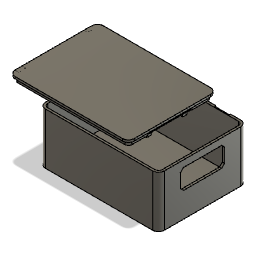
public-monitor-bridge-case (Autodesk Fusion 360 design; units mm, degrees)
Autodesk Fusion 360 part; units mm, degrees
note: some values were not read from the file. Set by a fixed rule: which face or edge a step refers to.
sketch "Base" plane through (0, 0, 0) normal (0, 1, 0) x (1, 0, 0) in component "Top"
  line L0 (0, 0) -> (81, 0)
  line L1 (81, 0) -> (81, 60)
  line L2 (81, 60) -> (0, 60)
  line L3 (0, 60) -> (0, 0)
  dimension "d6" = 81
  dimension "d7" = 60
  constraint horizontal L0
  constraint vertical L1
  constraint horizontal L2
  constraint vertical L3
  constraint coincident L0.start L3.end
  measures "d6" distance of L0.start L0.end
  measures "d7" distance of L0.start L2.end
extrude "Extrude1" add sketch "Base" along normal blind 35 makes body 1 in component "Top"
fillet "Fillet1" radius 4 4 edges at (81, 17.5, 0) (0, 17.5, 0) (81, 17.5, -60) (0, 17.5, -60) on bodies 1 in component "Top"
shell "Shell1" thickness 1.5 removed faces 1 at (52.6667, 35, -20) on bodies 1 in component "Top"
sketch "Knob" plane through (1.5, 0, 0) normal (1, 0, 0) x (0, 0, -1) in component "Top"
  line L0 (56, 1.5) -> (56, 35)
  line L1 (56, 35) -> (4, 35)
  line L2 (4, 35) -> (4, 1.5)
  line L3 (4, 1.5) -> (56, 1.5)
  line L4 (15, 35) -> (45, 35)
  line L5 (45, 35) -> (45, 32)
  line L6 (45, 32) -> (15, 32)
  line L7 (15, 32) -> (15, 35)
  line L8 (30, 35) -> (30, 32) construction
  dimension "d12" = 30
  dimension "d13" = 3
  constraint horizontal L4
  constraint vertical L5
  constraint horizontal L6
  constraint vertical L7
  constraint coincident L1 L4.start
  constraint midpoint L1 L8.start
  constraint midpoint L6 L8.end
  constraint vertical L8
  measures "d12" distance of L5.end L6.end
  measures "d13" distance of L4.end L5.end
extrude "Extrude2" add sketch "Knob" along normal blind 6 draft -45 contours L1 L4 L5 L6 L7 bodies 1 in component "Top"
ref_plane "WorkPlane2" through (40.5, 17.5, -30) normal (-1, 0, 0) x (0, 0, 1) in component "Top"
mirror "Mirror1" about plane through (40.5, 17.5, -30) normal (-1, 0, 0) of "Extrude2" in component "Top"
sketch "Top" plane through (0, 35, 0) normal (0, 1, 0) x (-1, 0, 0) in component "Base"
  line L0 (-81, -4) -> (-81, -56)
  arc A0 (-81, -56) -> (-77, -60) centre (-77, -56) ccw
  line L1 (-77, -60) -> (-4, -60)
  arc A1 (-4, -60) -> (0, -56) centre (-4, -56) ccw
  line L2 (0, -56) -> (0, -4)
  arc A2 (0, -4) -> (-4, 0) centre (-4, -4) ccw
  line L3 (-4, 0) -> (-77, 0)
  arc A3 (-77, 0) -> (-81, -4) centre (-77, -4) ccw
  line L4 (-79.5, -15) -> (-79.5, -4)
  arc A4 (-77, -1.5) -> (-79.5, -4) centre (-77, -4) ccw
  line L5 (-77, -1.5) -> (-4, -1.5)
  arc A5 (-1.5, -4) -> (-4, -1.5) centre (-4, -4) ccw
  line L6 (-1.5, -4) -> (-1.5, -15)
  line L7 (-1.5, -15) -> (-1.5, -45)
  line L8 (-1.5, -45) -> (-1.5, -56)
  arc A6 (-4, -58.5) -> (-1.5, -56) centre (-4, -56) ccw
  line L9 (-4, -58.5) -> (-77, -58.5)
  arc A7 (-79.5, -56) -> (-77, -58.5) centre (-77, -56) ccw
  line L10 (-79.5, -56) -> (-79.5, -45)
  line L11 (-79.5, -45) -> (-79.5, -15)
extrude "Extrude1'" add sketch "Top" along normal blind 1.5 separate body contours L0 A0 L1 A1 L2 A2 L3 A3 | L4 A4 L5 A5 L6 L7 L8 A6 L9 A7 L10 L11 makes body 2 in component "Base"
sketch "Lip" plane through (0, 35, 0) normal (0, -1, 0) x (1, 0, 0) in component "Base"
  arc A0 (81, -4) -> (77, 0) centre (77, -4) ccw
  line L0 (77, 0) -> (4, 0)
  arc A1 (4, 0) -> (0, -4) centre (4, -4) ccw
  line L1 (0, -4) -> (0, -56)
  arc A2 (0, -56) -> (4, -60) centre (4, -56) ccw
  line L2 (4, -60) -> (77, -60)
  arc A3 (77, -60) -> (81, -56) centre (77, -56) ccw
  line L3 (81, -56) -> (81, -4)
  line L4 (79.3, -56) -> (79.3, -4)
  arc A4 (79.3, -4) -> (77, -1.7) centre (77, -4) ccw
  line L5 (77, -1.7) -> (4, -1.7)
  arc A5 (4, -1.7) -> (1.7, -4) centre (4, -4) ccw
  line L6 (1.7, -4) -> (1.7, -56)
  arc A6 (1.7, -56) -> (4, -58.3) centre (4, -56) ccw
  line L7 (4, -58.3) -> (77, -58.3)
  arc A7 (77, -58.3) -> (79.3, -56) centre (77, -56) ccw
  dimension "d19" = 1.7
extrude "Extrude2'" add sketch "Lip" along normal blind 3 contours L4 A4 L5 A5 L6 A6 L7 A7 bodies 2 in component "Base"
extrude "Extrude3" cut sketch "Knob" along normal blind 3 draft -45 from surface at 0.2 contours L1 L4 L5 L6 L7 bodies 2 in component "Base"
mirror "Mirror1'" about plane through (40.5, 17.5, -30) normal (-1, 0, 0) of "Extrude3" in component "Base"
shell "Shell1'" thickness 1.5 removed faces 1 at (27.5667, 32, -35) on bodies 2 in component "Base"
chamfer "Chamfer1" distance 0.6 angle 45 2 edges at (1.7, 32, -30) (79.3, 32, -30) on bodies 2 in component "Base"
sketch "ttl-cutout" plane through (81, 0, 0) normal (1, 0, 0) x (0, 0, -1) in component "Top"
  line L0 (56, 35) -> (4, 35)
  line L1 (4, 35) -> (4, 0)
  line L2 (4, 0) -> (56, 0)
  line L3 (56, 0) -> (56, 35)
  line L4 (0, 35) -> (0, 0)
  line L5 (0, 0) -> (60, 0)
  line L6 (15, 35) -> (45, 35)
  line L7 (45, 35) -> (45, 17)
  line L8 (45, 17) -> (15, 17)
  line L9 (15, 17) -> (15, 35)
  line L10 (30, 35) -> (30, 0) construction
  line L11 (45, 35) -> (43.5, 33.5) construction
  line L12 (43.5, 33.5) -> (16.5, 33.5) construction
  line L13 (16.5, 33.5) -> (15, 35) construction
  line L14 (15, 35) -> (45, 35) construction
  line L15 (15, 32) -> (16.5, 33.5) construction
  line L16 (16.5, 33.5) -> (43.5, 33.5) construction
  line L17 (43.5, 33.5) -> (45, 32) construction
  line L18 (45, 32) -> (15, 32) construction
  line L19 (15, 30.5) -> (45, 30.5)
  point P0 (30, 17)
  point P1 (30, 35)
  dimension "d73" = 30
  dimension "d74" = 18
  dimension "d75" = 1.5
  constraint horizontal L6
  constraint vertical L7
  constraint horizontal L8
  constraint vertical L9
  constraint coincident L0 L6.start
  constraint midpoint L8 P0
  constraint midpoint L0 P1
  constraint coincident P1 L10.start
  constraint midpoint L2 L10.end
  constraint coincident P0 L10
  constraint coincident L9 L19.start
  constraint coincident L7 L19.end
  constraint perpendicular L7 L19
  measures "d73" distance of L6.start L6.end
  measures "d74" distance of L6.start L8.end
  measures "d75" distance of L18 L19
sketch "pcb-mount" plane through (12.1976, 35, -8.3625) normal (0, -1, 0) x (1, 0, 0) in component "Base"
  line L0 (66.5024, -7.2375) -> (67.1024, -6.6375)
  line L1 (67.1024, -6.6375) -> (67.1024, 4.3625)
  arc A0 (67.1024, 4.3625) -> (64.8024, 6.6625) centre (64.8024, 4.3625) ccw
  line L2 (64.8024, 6.6625) -> (-8.1976, 6.6625)
  arc A1 (-8.1976, 6.6625) -> (-10.4976, 4.3625) centre (-8.1976, 4.3625) ccw
  line L3 (-10.4976, 4.3625) -> (-10.4976, -6.6375)
  line L4 (-10.4976, -6.6375) -> (-9.8976, -7.2375)
  line L5 (-9.8976, -7.2375) -> (-9.8976, -36.0375)
  line L6 (-9.8976, -36.0375) -> (-10.4976, -36.6375)
  line L7 (-10.4976, -36.6375) -> (-10.4976, -47.6375)
  arc A2 (-10.4976, -47.6375) -> (-8.1976, -49.9375) centre (-8.1976, -47.6375) ccw
  line L8 (-8.1976, -49.9375) -> (64.8024, -49.9375)
  arc A3 (64.8024, -49.9375) -> (67.1024, -47.6375) centre (64.8024, -47.6375) ccw
  line L9 (67.1024, -47.6375) -> (67.1024, -36.6375)
  line L10 (67.1024, -36.6375) -> (66.5024, -36.0375)
  line L11 (66.5024, -36.0375) -> (66.5024, -7.2375)
  line L12 (64.8024, -48.4375) -> (-8.1976, -48.4375)
  arc A4 (-8.9976, -47.6375) -> (-8.1976, -48.4375) centre (-8.1976, -47.6375) ccw
  line L13 (-8.9976, -47.6375) -> (-8.9976, -37.2588)
  line L14 (-8.9976, -37.2588) -> (-8.3762, -36.6375)
  line L15 (-8.3762, -36.6375) -> (-8.3762, -6.6375)
  line L16 (-8.3762, -6.6375) -> (-8.9976, -6.0162)
  line L17 (-8.9976, -6.0162) -> (-8.9976, 4.3625)
  arc A5 (-8.1976, 5.1625) -> (-8.9976, 4.3625) centre (-8.1976, 4.3625) ccw
  line L18 (-8.1976, 5.1625) -> (64.8024, 5.1625)
  arc A6 (65.6024, 4.3625) -> (64.8024, 5.1625) centre (64.8024, 4.3625) ccw
  line L19 (65.6024, 4.3625) -> (65.6024, -6.0162)
  line L20 (65.6024, -6.0162) -> (64.9811, -6.6375)
  line L21 (64.9811, -6.6375) -> (64.9811, -36.6375)
  line L22 (64.9811, -36.6375) -> (65.6024, -37.2588)
  line L23 (65.6024, -37.2588) -> (65.6024, -47.6375)
  arc A7 (64.8024, -48.4375) -> (65.6024, -47.6375) centre (64.8024, -47.6375) ccw
  line L24 (6.6308, -40.2034) -> (6.6308, -39.4472)
  arc A8 (6.874, -39.1877) -> (6.6308, -39.4472) centre (6.8908, -39.4472) ccw
  line L25 (26.7308, -0.2034) -> (26.7308, -40.2034)
  line L26 (-4.5692, -0.2034) -> (26.7308, -0.2034)
  line L27 (-1.5692, -33.2034) -> (-4.5692, -33.2034)
  line L28 (-4.5692, -0.2034) -> (26.7308, -40.2034) construction
  arc A9 (13.8276, -38.8086) -> (13.6461, -38.7503) centre (13.6628, -39.0097) ccw
  line L29 (15.5308, -40.2034) -> (13.8276, -38.8086)
  line L30 (-1.5692, -40.2034) -> (-1.5692, -33.2034)
  line L31 (6.874, -39.1877) -> (13.6461, -38.7503)
  line L32 (-4.5692, -40.2034) -> (26.7308, -0.2034) construction
  line L33 (-1.5692, -0.2034) -> (-4.526, -3.2031)
  line L34 (11.0808, -0.2034) -> (11.0808, -40.2034) construction
  line L35 (26.7308, -40.2034) -> (-4.5692, -40.2034)
  line L36 (-4.5692, -40.2034) -> (-4.5692, -0.2034)
  line L37 (35.1346, -5.8875) -> (63.6346, -5.8875)
  line L38 (63.6346, -5.8875) -> (63.6346, -37.3875)
  line L39 (63.6346, -37.3875) -> (35.1346, -37.3875)
  line L40 (35.1346, -37.3875) -> (35.1346, -5.8875)
  line L41 (34.9346, -5.6875) -> (63.8346, -5.6875)
  line L42 (63.8346, -5.6875) -> (63.8346, -37.5875)
  line L43 (63.8346, -37.5875) -> (34.9346, -37.5875)
  line L44 (34.9346, -37.5875) -> (34.9346, -5.6875)
  line L45 (33.7346, -4.4875) -> (65.0346, -4.4875)
  line L46 (65.0346, -4.4875) -> (65.0346, -38.7875)
  line L47 (65.0346, -38.7875) -> (33.7346, -38.7875)
  line L48 (33.7346, -38.7875) -> (33.7346, -4.4875)
  line L49 (-5.9692, 1.1966) -> (28.1308, 1.1966)
  line L50 (28.1308, 1.1966) -> (28.1308, -41.6034)
  line L51 (28.1308, -41.6034) -> (-5.9692, -41.6034)
  line L52 (-5.9692, -41.6034) -> (-5.9692, 1.1966)
  line L53 (-4.7692, -0.0034) -> (26.9308, -0.0034)
  line L54 (26.9308, -0.0034) -> (26.9308, -40.4034)
  line L55 (26.9308, -40.4034) -> (-4.7692, -40.4034)
  line L56 (-4.7692, -40.4034) -> (-4.7692, -0.0034)
  line L57 (64.9811, -21.6375) -> (-8.3762, -21.6375) construction
  arc A10 (64.8024, -48.4375) -> (65.6024, -47.6375) centre (64.8024, -47.6375) ccw
  line L58 (65.6024, -47.6375) -> (65.6024, -37.2588)
  line L59 (65.6024, -37.2588) -> (64.9811, -36.6375)
  line L60 (64.9811, -36.6375) -> (64.9811, -6.6375)
  line L61 (64.9811, -6.6375) -> (65.6024, -6.0162)
  line L62 (65.6024, -6.0162) -> (65.6024, 4.3625)
  arc A11 (65.6024, 4.3625) -> (64.8024, 5.1625) centre (64.8024, 4.3625) ccw
  line L63 (64.8024, 5.1625) -> (-8.1976, 5.1625)
  arc A12 (-8.1976, 5.1625) -> (-8.9976, 4.3625) centre (-8.1976, 4.3625) ccw
  line L64 (-8.9976, 4.3625) -> (-8.9976, -6.0162)
  line L65 (-8.9976, -6.0162) -> (-8.3762, -6.6375)
  line L66 (-8.3762, -6.6375) -> (-8.3762, -36.6375)
  line L67 (-8.3762, -36.6375) -> (-8.9976, -37.2588)
  line L68 (-8.9976, -37.2588) -> (-8.9976, -47.6375)
  arc A13 (-8.9976, -47.6375) -> (-8.1976, -48.4375) centre (-8.1976, -47.6375) ccw
  line L69 (-8.1976, -48.4375) -> (64.8024, -48.4375)
  line L70 (-4.526, -3.2031) -> (-1.5692, -0.2034)
  line L71 (-4.5692, -0.2034) -> (-4.526, -3.2031)
  line L72 (26.7308, -3.205) -> (23.7308, -0.2034)
  point P0 (6.6308, -40.2034)
  point P1 (6.6308, -39.2034)
  point P2 (15.5308, -40.2034)
  point P3 (-4.5692, -33.2034)
  point P4 (11.0808, -20.2034)
  point P5 (-1.5692, -40.2034)
  point P6 (26.6876, -3.2031)
  point P7 (23.7308, -0.2034)
  point P8 (63.8346, -21.6375)
  point P9 (64.9811, -21.6375)
  dimension "d54" = 40
  dimension "d55" = 31.3
  dimension "d56" = 3
  dimension "d57" = 3
  dimension "d58" = 7
  dimension "d59" = 3
  dimension "d60" = 4.45
  dimension "d61" = 1
  dimension "d62" = 4.45
  dimension "d63" = 0.26
  dimension "d64" = 0.26
  dimension "d65" = 28.5
  dimension "d66" = 31.5
  dimension "d67" = -0.2
  dimension "d68" = -1.4
  dimension "d69" = -1.4
  dimension "d70" = -0.2
  dimension "d95" = 20.0784
  constraint perpendicular L26 L36
  constraint parallel L25 L36
  constraint parallel L26 L35
  constraint coincident P4 L32
  constraint coincident P4 L28
  constraint midpoint L34.start L26
  constraint midpoint L34.end L35
  constraint coincident P7 L26
  constraint coincident P5 L35
  constraint coincident P3 L36
  constraint coincident P5 L30.start
  constraint perpendicular L30 L35
  constraint coincident P3 L27.end
  constraint perpendicular L27 L36
  constraint coincident P0 L35
  constraint coincident P0 L24.start
  constraint perpendicular L24 L35
  constraint coincident P2 L35
  constraint symmetric P0 P2 L34
  constraint tangent A9 L31
  constraint tangent A9 L29
  constraint coincident P1 L31
  constraint coincident P1 L24
  constraint tangent A8 L31
  constraint tangent L24 A8
  constraint horizontal L37
  constraint vertical L38
  constraint horizontal L39
  constraint vertical L40
  constraint midpoint L42 P8
  constraint midpoint L21 P9
  constraint coincident P9 L57.start
  constraint midpoint L15 L57.end
  constraint coincident P8 L57
  constraint parallel L33 L70
  constraint coincident L25 L72.start
  constraint coincident P7 L72.end
  measures "d54" distance of L25.start L25.end
  measures "d55" distance of L26.start L25.start
  measures "d56" distance of L25.start P6
  measures "d57" distance of L25.start P7
  measures "d58" distance of P3 L35
  measures "d59" distance of L32.start P5
  measures "d60" distance of P0 L34.end
  measures "d61" distance of P0 P1
  measures "d62" distance of P2 L34.end
  measures "d63" radius of A9
  measures "d64" radius of A8
  measures "d65" distance of L37.start L37.end
  measures "d66" distance of L37.start L39.end
  measures "d95" distance of L13 L34
extrude "Extrude6" add sketch "pcb-mount" along normal blind 6 contours L49 L50 L51 L52 bodies 2 in component "Base"
extrude "Extrude5" cut sketch "ttl-cutout" against normal up to surface (1.5 mm away) contours L7 L8 L9 L19 bodies 1 in component "Top"
chamfer "Chamfer1'" distance 2 angle 45 4 edges at (80.25, 30.5, -15) (80.25, 30.5, -45) (80.25, 17, -15) (80.25, 17, -45) on bodies 1 in component "Top"
sketch "makers-mark" plane through (40.5, 0, -30) normal (0, 1, 0) x (1, 0, 0) in component "Top"
extrude "Extrude11" add sketch "pcb-mount" along normal blind 4 contours L20 L21 L22 L45 L46 L47 L48 L59 L60 L61 | L20 L21 L22 L46 L59 L60 L61 bodies 2 in component "Base"
extrude "Extrude12" add sketch "pcb-mount" along normal up to surface (1.25 mm away) contours L37 L38 L39 L40 bodies 2 in component "Base"
sketch "usb-cutout" plane through (0, 0, -60) normal (0, 0, -1) x (-1, 0, 0) in component "Top"
  line L0 (-4, 0) -> (-4, 35)
  line L1 (-4, 35) -> (-77, 35)
  line L2 (-77, 35) -> (-77, 0)
  line L3 (-77, 0) -> (-4, 0)
  line L4 (-1.5, 1.5) -> (-4, 1.5)
  line L5 (-1.5, 1.5) -> (-4, 1.5)
  line L6 (-4, 1.5) -> (-77, 1.5)
  line L7 (-77, 1.5) -> (-79.5, 1.5)
  line L8 (-77, 1.5) -> (-79.5, 1.5)
  line L9 (-77, 1.5) -> (-4, 1.5)
  line L10 (-4, 1.5) -> (-4, 35) construction
  line L11 (-30, 31.5) -> (-18, 31.5)
  line L12 (-18, 31.5) -> (-18, 25.5)
  line L13 (-18, 25.5) -> (-30, 25.5)
  line L14 (-30, 25.5) -> (-30, 31.5)
  point P0 (-24, 31.5)
  dimension "d96" = 12
  dimension "d97" = 20
  dimension "d98" = 6
  dimension "d99" = 3.5
  constraint coincident L4.end L5.end
  constraint coincident L0.end L1.start
  constraint horizontal L11
  constraint vertical L12
  constraint horizontal L13
  constraint vertical L14
  constraint midpoint L11 P0
  measures "d96" distance of L11.start L11.end
  measures "d97" distance of L10 P0
  measures "d98" distance of L11.end L12.end
  measures "d99" distance of L1 L11
extrude "Extrude7" cut sketch "usb-cutout" against normal up to surface (1.5 mm away) contours L11 L12 L13 L14 bodies 1 in component "Top"
chamfer "Chamfer2" distance 1 angle 45 4 edges at (24, 25.5, -60) (30, 28.5, -60) (24, 31.5, -60) (18, 28.5, -60) on bodies 1 in component "Top"
chamfer "Chamfer3" distance 0.5 angle 45 4 edges at (24, 25.5, -58.5) (30, 28.5, -58.5) (24, 31.5, -58.5) (18, 28.5, -58.5) on bodies 1 in component "Top"
sketch "easy-open-notch" plane through (0, 0, -60) normal (0, 0, -1) x (-1, 0, 0) in component "Top"
  line L0 (-4, 0) -> (-4, 35)
  line L1 (-4, 35) -> (-77, 35)
  line L2 (-77, 35) -> (-77, 0)
  line L3 (-77, 0) -> (-4, 0)
  line L4 (-31, 24.5) -> (-31, 32.5)
  line L5 (-31, 32.5) -> (-17, 32.5)
  line L6 (-17, 32.5) -> (-17, 24.5)
  line L7 (-17, 24.5) -> (-31, 24.5)
  line L8 (-70, 35) -> (-60, 35)
  line L9 (-60, 35) -> (-60, 32)
  line L10 (-60, 32) -> (-70, 32)
  line L11 (-70, 32) -> (-70, 35)
  dimension "d104" = 10
  dimension "d105" = 3
  constraint horizontal L8
  constraint vertical L9
  constraint horizontal L10
  constraint vertical L11
  constraint coincident L1 L8.start
  measures "d104" distance of L8.start L8.end
  measures "d105" distance of L8.start L10.end
extrude "Extrude8" cut sketch "easy-open-notch" against normal blind 0.8 contours L1 L8 L9 L10 L11 bodies 1 in component "Top"
sketch "Sketch5" plane through (0, 31, 0) normal (0, -1, 0) x (1, 0, 0) in component "Base"
  line L0 (76.0322, -45.95) -> (47.1322, -45.95)
  line L1 (47.1322, -45.95) -> (47.1322, -14.05)
  line L2 (47.1322, -14.05) -> (76.0322, -14.05)
  line L3 (76.0322, -14.05) -> (76.0322, -45.95)
  line L4 (45.9322, -47.15) -> (77.2322, -47.15)
  line L5 (77.2322, -47.15) -> (77.2322, -12.85)
  line L6 (77.2322, -12.85) -> (45.9322, -12.85)
  line L7 (45.9322, -12.85) -> (45.9322, -47.15)
  line L8 (76.0322, -14.05) -> (76.0322, -12.85)
  line L9 (76.0322, -45.95) -> (76.0322, -47.15)
  constraint coincident L2.end L3.start
  constraint coincident L6 L8.end
  constraint perpendicular L6 L8
  constraint coincident L0.start L3.end
  constraint coincident L4 L9.end
  constraint perpendicular L4 L9
extrude "Extrude13" add sketch "Sketch5" along normal blind 2 contours L0 L1 L2 L4 L6 L7 L8 L9 bodies 2 in component "Base"
sketch "Sketch6" plane through (0, 0, -14.05) normal (0, 0, -1) x (-1, 0, 0) in component "Base"
  line L0 (-47.1322, 35) -> (-76.0322, 35)
  line L1 (-76.0322, 35) -> (-76.0322, 31)
  line L2 (-76.0322, 31) -> (-76.0322, 29)
  line L3 (-76.0322, 29) -> (-47.1322, 29)
  line L4 (-47.1322, 29) -> (-47.1322, 35)
  line L5 (-56.5322, 29) -> (-68.5322, 29)
  line L6 (-68.5322, 29) -> (-68.5322, 30.5)
  line L7 (-68.5322, 30.5) -> (-56.5322, 30.5)
  line L8 (-56.5322, 30.5) -> (-56.5322, 29)
  dimension "d110" = 1.5
  dimension "d115" = 12
  dimension "d116" = 7.5
  constraint horizontal L5
  constraint vertical L6
  constraint horizontal L7
  constraint vertical L8
  constraint coincident L3 L5.start
  measures "d110" distance of L5.start L7.end
  measures "d115" distance of L5.start L5.end
  measures "d116" distance of L2 L6
extrude "Extrude14" add sketch "Sketch6" along normal blind 1.5 draft -45 contours L3 L5 L6 L7 L8 bodies 2 in component "Base"
sketch "Sketch8" plane through (0, 0, -8.366) normal (0, 0, -1) x (-1, 0, 0) in component "Base"
  line L0 (-7.4284, 35) -> (-39.1284, 35)
  line L1 (-39.1284, 35) -> (-39.1284, 29)
  line L2 (-39.1284, 29) -> (-7.4284, 29)
  line L3 (-7.4284, 29) -> (-7.4284, 35)
  line L4 (-17.1836, 29) -> (-29.1836, 29)
  line L5 (-29.1836, 29) -> (-29.1836, 30.5)
  line L6 (-29.1836, 30.5) -> (-17.1836, 30.5)
  line L7 (-17.1836, 30.5) -> (-17.1836, 29)
  point P0 (-23.1836, 30.5)
  dimension "d117" = 12
  dimension "d118" = 1.5
  constraint horizontal L4
  constraint vertical L5
  constraint horizontal L6
  constraint vertical L7
  constraint coincident L2 L4.start
  constraint midpoint L6 P0
  measures "d117" distance of L4.start L4.end
  measures "d118" distance of L4.start L6.end
extrude "Extrude15" add sketch "Sketch8" along normal blind 1.75 draft -30 contours L2 L4 L5 L6 L7 bodies 2 in component "Base"
sketch "Sketch9" plane through (7.4284, 0, 0) normal (1, 0, 0) x (0, 0, -1) in component "Base"
  line L0 (48.766, 35) -> (8.366, 35)
  line L1 (8.366, 35) -> (8.366, 29)
  line L2 (8.366, 29) -> (48.766, 29)
  line L3 (48.766, 29) -> (48.766, 35)
  line L4 (35.1023, 29) -> (23.1023, 29)
  line L5 (23.1023, 29) -> (23.1023, 30.5)
  line L6 (23.1023, 30.5) -> (35.1023, 30.5)
  line L7 (35.1023, 30.5) -> (35.1023, 29)
  dimension "d121" = 12
  dimension "d122" = 1.5
  constraint horizontal L4
  constraint vertical L5
  constraint horizontal L6
  constraint vertical L7
  constraint coincident L2 L4.start
  measures "d121" distance of L4.start L4.end
  measures "d122" distance of L4.start L6.end
extrude "Extrude16" add sketch "Sketch9" along normal blind 1.75 draft -35 contours L2 L4 L5 L6 L7 bodies 2 in component "Base"
sketch "Sketch12" plane through (39.1284, 0, 0) normal (-1, 0, 0) x (0, 0, 1) in component "Base"
  line L0 (-8.366, 35) -> (-48.766, 35)
  line L1 (-48.766, 35) -> (-48.766, 29)
  line L2 (-48.766, 29) -> (-8.366, 29)
  line L3 (-8.366, 29) -> (-8.366, 35)
  line L4 (-35.8969, 29) -> (-23.8969, 29)
  line L5 (-23.8969, 29) -> (-23.8969, 30.5)
  line L6 (-23.8969, 30.5) -> (-35.8969, 30.5)
  line L7 (-35.8969, 30.5) -> (-35.8969, 29)
  point P0 (-29.8969, 30.5)
  dimension "d129" = 12
  dimension "d130" = 1.5
  constraint horizontal L4
  constraint vertical L5
  constraint horizontal L6
  constraint vertical L7
  constraint coincident L2 L4.start
  constraint midpoint L6 P0
  measures "d129" distance of L5.end L6.end
  measures "d130" distance of L4.start L6.end
extrude "Extrude17" add sketch "Sketch12" along normal blind 1.5 draft -45 contours L2 L4 L5 L6 L7 bodies 2 in component "Base"
sketch "Sketch13" plane through (0, 0, 0) normal (-1, 0, 0) x (0, 0, 1) in component "Base"
  line L0 (-56, 35) -> (-4, 35)
  line L1 (-4, 35) -> (-4, 36.5)
  line L2 (-4, 36.5) -> (-56, 36.5)
  line L3 (-56, 36.5) -> (-56, 35)
  line L4 (-56, 35) -> (-51, 35)
  line L5 (-51, 35) -> (-51, 36)
  line L6 (-51, 36) -> (-56, 36)
  line L7 (-56, 36) -> (-56, 35)
  line L8 (-4, 35) -> (-9, 35)
  line L9 (-9, 35) -> (-9, 36)
  line L10 (-9, 36) -> (-4, 36)
  line L11 (-4, 36) -> (-4, 35)
  dimension "d131" = 5
  dimension "d132" = 5
  dimension "d133" = 1
  dimension "d134" = 1
  constraint horizontal L4
  constraint vertical L5
  constraint horizontal L6
  constraint vertical L7
  constraint coincident L0.start L3.end
  constraint horizontal L8
  constraint vertical L9
  constraint horizontal L10
  constraint vertical L11
  constraint coincident L0.end L1.start
  measures "d131" distance of L0.start L4.end
  measures "d132" distance of L0.end L8.end
  measures "d133" distance of L8.end L9.end
  measures "d134" distance of L0.start L6.end
extrude "Extrude18" cut sketch "Sketch13" against normal up to surface (2.3 mm away) contours L0 L3 L4 L5 L6 L7 | L0 L1 L8 L9 L10 L11 bodies 2 in component "Base"
sketch "Sketch14" plane through (0, 0, -49.966) normal (0, 0, -1) x (-1, 0, 0) in component "Base"
  line L0 (-6.2284, 35) -> (-40.3284, 35)
  line L1 (-40.3284, 35) -> (-40.3284, 29)
  line L2 (-40.3284, 29) -> (-6.2284, 29)
  line L3 (-6.2284, 29) -> (-6.2284, 35)
  line L4 (-18.9172, 35) -> (-18.9172, 28.9971)
  line L5 (-28.1205, 35) -> (-28.1205, 28.9999)
  line L6 (-77, 32) -> (-4, 32)
  line L7 (-40.3284, 35) -> (-6.2284, 35)
  line L8 (-4, 32) -> (-77, 32)
  line L9 (-18.9172, 31.9986) -> (-28.1205, 31.9999)
  constraint vertical L4
  constraint coincident L0 L4.start
  constraint vertical L5
  constraint coincident L0 L5.start
  constraint midpoint L4 L9.start
  constraint midpoint L5 L9.end
extrude "Extrude20" cut sketch "Sketch14" against normal up to surface (1.2 mm away) contours L2 L4 L5 L6 L8 L9 bodies 2 in component "Base"
extrude "Extrude19" cut sketch "Sketch14" against normal up to surface (1.2 mm away) contours L2 L4 L5 L6 L8 L9 bodies 2 in component "Base"
extrude "Extrude21" add sketch "pcb-mount" along normal blind 1 contours L24 A8 L25 L26 L27 A9 L29 L30 L31 L33 L35 L36 L70 L71 L72 bodies 2 in component "Base"
sketch "Sketch15" plane through (0, 31, 0) normal (0, -1, 0) x (1, 0, 0) in component "Base"
  line L0 (76.0322, -12.85) -> (76.0322, -14.05)
  line L1 (76.0322, -14.05) -> (76.0322, -45.95)
  line L2 (76.0322, -45.95) -> (76.0322, -47.15)
  line L3 (76.0322, -47.15) -> (77.2322, -47.15)
  line L4 (77.2322, -47.15) -> (77.2322, -12.85)
  line L5 (77.2322, -12.85) -> (76.0322, -12.85)
  line L6 (76.0322, -43.65) -> (77.2322, -43.65)
  line L7 (77.2322, -43.65) -> (77.2322, -40.65)
  line L8 (77.2322, -40.65) -> (76.0322, -40.65)
  line L9 (76.0322, -40.65) -> (76.0322, -43.65)
  line L10 (76.0322, -30) -> (77.2322, -30) construction
  line L11 (76.0322, -16.35) -> (77.2322, -16.35)
  line L12 (76.0322, -19.35) -> (76.0322, -16.35)
  line L13 (77.2322, -19.35) -> (76.0322, -19.35)
  line L14 (77.2322, -16.35) -> (77.2322, -19.35)
  dimension "d145" = 3
  dimension "d146" = 2.3
  constraint horizontal L6
  constraint vertical L7
  constraint horizontal L8
  constraint vertical L9
  constraint coincident L4 L7.end
  constraint coincident L1 L6.start
  constraint midpoint L1 L10.start
  constraint midpoint L4 L10.end
  constraint symmetric L6.start L10 L11.start
  constraint symmetric L6.end L10 L11.end
  constraint symmetric L7.end L10 L13.start
  constraint symmetric L8.end L10 L12.start
  measures "d145" distance of L6.start L8.end
  measures "d146" distance of L1.end L6.start
extrude "Extrude22" add sketch "Sketch15" along normal up to surface (2 mm away) contours L1 L4 L11 L12 L13 L14 | L1 L4 L6 L7 L8 L9 bodies 2 in component "Base"
sketch "Sketch16" plane through (0, 0, -14.05) normal (0, 0, -1) x (1, 0, 0) in component "Base"
sketch "Sketch17" plane through (47.1322, 0, 0) normal (1, 0, 0) x (0, 0, -1) in component "Base"
  line L0 (45.95, 35) -> (14.05, 35)
  line L1 (14.05, 35) -> (14.05, 29)
  line L2 (14.05, 29) -> (45.95, 29)
  line L3 (45.95, 29) -> (45.95, 35)
  line L4 (36, 30.5) -> (36, 29)
  line L5 (24, 29) -> (24, 30.5)
  line L6 (24, 30.5) -> (36, 30.5)
  line L7 (36, 29) -> (24, 29)
  point P0 (30, 29)
  point P1 (30, 29)
  dimension "d149" = 1.5
  dimension "d150" = 12
  constraint horizontal L7
  constraint vertical L5
  constraint horizontal L6
  constraint vertical L4
  constraint midpoint L2 P1
  constraint midpoint L7 P1
  constraint coincident P1 P0
  measures "d149" distance of L4.start L4.end
  measures "d150" distance of L5.start L4.end
sketch "Sketch18" plane through (0, 0, -45.95) normal (0, 0, 1) x (1, 0, 0) in component "Base"
  line L0 (76.0322, 35) -> (47.1322, 35)
  line L1 (47.1322, 35) -> (47.1322, 29)
  line L2 (47.1322, 29) -> (76.0322, 29)
  line L3 (76.0322, 29) -> (76.0322, 31)
  line L4 (76.0322, 31) -> (76.0322, 35)
  line L5 (57.2822, 29.75) -> (67.7822, 29.75)
  line L6 (67.7822, 29.75) -> (68.5322, 29)
  line L7 (68.5322, 29) -> (56.5322, 29)
  line L8 (56.5322, 29) -> (57.2822, 29.75)
  line L9 (57.2822, 29.75) -> (67.7822, 29.75)
  line L10 (57.2822, 29.75) -> (56.5322, 30.5)
  line L11 (56.5322, 30.5) -> (68.5322, 30.5)
  line L12 (68.5322, 30.5) -> (67.7822, 29.75)
  line L13 (67.7822, 29.75) -> (57.2822, 29.75)
  line L14 (56.5322, 30.5) -> (57.2822, 29.75)
  line L15 (57.2822, 29.75) -> (56.5322, 29)
  line L16 (56.5322, 29) -> (56.5322, 30.5)
  line L17 (68.5322, 29) -> (67.7822, 29.75)
  line L18 (67.7822, 29.75) -> (68.5322, 30.5)
  line L19 (68.5322, 30.5) -> (68.5322, 29)
extrude "Extrude23" add sketch "Sketch18" along normal blind 1.5 draft -45 contours L2 L5 L6 L7 L8 L9 L13 L15 L17 | L8 L10 L14 L15 L16 | L6 L12 L17 L18 L19 | L5 L9 L10 L11 L12 L13 L14 L18 bodies 2 in component "Base"
extrude "Extrude24" add sketch "Sketch17" along normal blind 1.5 draft -45 contours L2 L4 L5 L6 L7 bodies 2 in component "Base"
component "Enclosure" placed x (1, 0, 0) y (0, 1, 0) z (0, 0, 1) at (0, 0, 0)
component "Top" placed x (1, 0, 0) y (0, 1, 0) z (0, 0, 1) at (0, 0, 0) in component "Enclosure"
component "Base" placed x (1, 0, 0) y (0, 1, 0) z (0, 0, 1) at (-12.1976, 15.6554, 8.3625) in component "Enclosure"
equation "Width = 60 mm"
equation "length = 81 mm"
equation "heigth = 35 mm"
equation "shell = 1.5 mm"
equation "gap = 0.2 mm"
equation "d6 = length"
equation "d7 = Width"
equation "d8 = heigth"
equation "d11 = shell"
equation "d12 = Width / 2"
equation "d13 = shell * 2"
equation "d17 = shell"
equation "d19 = shell + gap"
equation "d20 = shell * 2"
equation "d23 = shell * 2"
equation "d26 = shell"
equation "d57 = d155"
equation "d60 = ( 8.9 / 2 ) * 1 mm"
equation "d62 = d159"
equation "d65 = 32.5 mm - 4 mm"
equation "d134 = d133"
equation "d152 = 45 deg - 45 deg - 45 deg"
